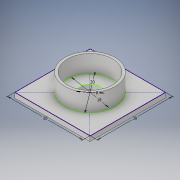
# Autodesk Inventor part: RodamientoAspa
Saved by Autodesk Inventor 2019 (Build 230136000, 136)
## iProperties
Created: 2018-08-28
Part Number: RodamientoAspa
Material: Genérico
Document SubType Name: Modeling
Designer: Cecilia Barrera Vill
Density: 1 g/cm^3
Appearance: Valor por defecto
Author: Cecilia Barrera Vill
Autodesk Inventor part; units mm, degrees
ref_plane "YZ Plane" through (0, 0, 0) normal (1, 0, 0) x (0, 1, 0)
ref_plane "XZ Plane" through (0, 0, 0) normal (0, 1, 0) x (-1, 0, 0)
ref_plane "XY Plane" through (0, 0, 0) normal (0, 0, 1) x (1, 0, 0)
sketch "Boceto1" plane through (0, 0, 0) normal (0, 1, 0) x (-1, 0, 0)
  line L0 (15, -15) -> (-15, -15)
  line L1 (-15, -15) -> (-15, 15)
  line L2 (-15, 15) -> (15, 15)
  line L3 (15, 15) -> (15, -15)
  line L4 (15, -15) -> (-15, 15) construction
  line L5 (-15, -15) -> (15, 15) construction
  circle A0 centre (0, 0) radius 9
  circle A1 centre (0, 0) radius 4
  circle A2 centre (0, 0) radius 10
  dimension "d0" = 30
  dimension "d1" = 30
  dimension "d9" = 18
  dimension "d12" = 8
  dimension "d15" = 20
  constraints: 12 end point, 3 centre point, 2 coincident, 2 midpoint, 2 parallel, 1 horizontal, 1 perpendicular
  measures "d0" distance of L1.end L2.end
  measures "d1" distance of L0.end L1.end
  measures "d9" diameter of A0
  measures "d12" diameter of A1
  measures "d15" diameter of A2
extrude "Extrusión1" add sketch "Boceto1" against normal blind 2 contours L0 L1 L2 L3 | A0 | A1 | A2
extrude "Extrusión4" cut sketch "Boceto1" against normal blind 3 contours A1
extrude "Extrusión5" add sketch "Boceto1" along normal blind 7 contours A2
